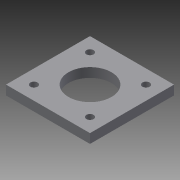
# Autodesk Inventor part: BallBearingHolderOutside
Saved by Autodesk Inventor 2015 (Build 190159000, 159)
## iProperties
Created: 2017-03-08
Part Number: BallBearingHolderOutside
Material: Generic
Document SubType Name: Modeling
Designer: Ernest
Density: 1 g/cm^3
Appearance: Default
Author: Ernest
Autodesk Inventor part; units mm, degrees
ref_plane "YZ Plane" through (0, 0, 0) normal (1, 0, 0) x (0, 1, 0)
ref_plane "XZ Plane" through (0, 0, 0) normal (0, 1, 0) x (-1, 0, 0)
ref_plane "XY Plane" through (0, 0, 0) normal (0, 0, 1) x (1, 0, 0)
sketch "Sketch1" plane through (0, 0, 0) normal (0, 0, 1) x (1, 0, 0)
  circle A0 centre (0, 0) radius 11.5
  circle A1 centre (0, 0) radius 14.3 construction
  line L0 (-22.5, 22.5) -> (22.5, 22.5)
  line L1 (22.5, 22.5) -> (22.5, -22.5)
  line L2 (22.5, -22.5) -> (-22.5, -22.5)
  line L3 (-22.5, -22.5) -> (-22.5, 22.5)
  line L4 (-15, 15) -> (15, 15) construction
  line L5 (15, 15) -> (15, -15) construction
  line L6 (15, -15) -> (-15, -15) construction
  line L7 (-15, -15) -> (-15, 15) construction
  line L8 (-11.6401, 18.3599) -> (-10.4103, 13.7702)
  line L9 (-10.4103, 13.7702) -> (-13.7702, 10.4103)
  line L10 (-13.7702, 10.4103) -> (-18.3599, 11.6401)
  line L11 (-18.3599, 11.6401) -> (-19.5897, 16.2298)
  line L12 (-19.5897, 16.2298) -> (-16.2298, 19.5897)
  line L13 (-16.2298, 19.5897) -> (-11.6401, 18.3599)
  line L14 (18.3599, 11.6401) -> (13.7702, 10.4103)
  line L15 (13.7702, 10.4103) -> (10.4103, 13.7702)
  line L16 (10.4103, 13.7702) -> (11.6401, 18.3599)
  line L17 (11.6401, 18.3599) -> (16.2298, 19.5897)
  line L18 (16.2298, 19.5897) -> (19.5897, 16.2298)
  line L19 (19.5897, 16.2298) -> (18.3599, 11.6401)
  line L20 (18.3599, -11.6401) -> (19.5897, -16.2298)
  line L21 (19.5897, -16.2298) -> (16.2298, -19.5897)
  line L22 (16.2298, -19.5897) -> (11.6401, -18.3599)
  line L23 (11.6401, -18.3599) -> (10.4103, -13.7702)
  line L24 (10.4103, -13.7702) -> (13.7702, -10.4103)
  line L25 (13.7702, -10.4103) -> (18.3599, -11.6401)
  line L26 (-18.3599, -11.6401) -> (-13.7702, -10.4103)
  line L27 (-13.7702, -10.4103) -> (-10.4103, -13.7702)
  line L28 (-10.4103, -13.7702) -> (-11.6401, -18.3599)
  line L29 (-11.6401, -18.3599) -> (-16.2298, -19.5897)
  line L30 (-16.2298, -19.5897) -> (-19.5897, -16.2298)
  line L31 (-19.5897, -16.2298) -> (-18.3599, -11.6401)
  line L32 (-15, 15) -> (15, -15) construction
  line L33 (15, 15) -> (-15, -15) construction
  circle A2 centre (-15, 15) radius 1.95
  circle A3 centre (15, 15) radius 1.95
  circle A4 centre (15, -15) radius 1.95
  circle A5 centre (-15, -15) radius 1.95
  dimension "d0" = 28.6
  dimension "d1" = 23
  dimension "d6" = 8.23
  dimension "d7" = 30
  dimension "d8" = 30
  dimension "d9" = 3.9
  dimension "d10" = 45
  dimension "d11" = 22.5
  dimension "d12" = 45
  dimension "d13" = 22.5
  constraints: 68 end point, 10 coincident, 6 centre point, 6 perpendicular, 4 parallel, 3 equal length, 3 equal radius, 2 horizontal, 2 midpoint, 52 other
  measures "d0" diameter of A1
  measures "d1" diameter of A0
  measures "d6" distance between parallel lines of L10 L13
  measures "d7" distance of L4.start L4.end
  measures "d8" distance of L6.end L4.start
  measures "d9" diameter of A2
  measures "d10" distance of L1.end L2.end
  measures "d11" distance from line of point (0, 0) L3
  measures "d12" distance of L0.end L1.end
  measures "d13" distance from line of point (0, 0) L0
extrude "Extrusion3" add sketch "Sketch1" along normal blind 5 contours L0 L1 L2 L3 | L8 L9 L10 L11 L12 L13 | L14 L15 L16 L17 L18 L19 | L20 L21 L22 L23 L24 L25 | L26 L27 L28 L29 L30 L31
extrude "Extrusion4" cut sketch "Sketch1" along normal blind 2.5 contours L8 L9 L10 L11 L12 L13 | L14 L15 L16 L17 L18 L19 | L20 L21 L22 L23 L24 L25 | L26 L27 L28 L29 L30 L31
equation "\"d11\" = 0.5 * d10"
equation "\"d13\" = 0.5 * d12"
body "Solid2"
